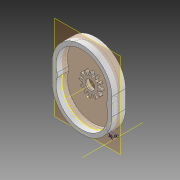
# Autodesk Inventor part: housing
Saved by Autodesk Inventor 2020 (Build 240168000, 168)
## iProperties
Created: 2020-11-24
Part Number: housing
Material: Generic
Document SubType Name: Modeling
Designer: DDeGo
Density: 1 g/cm^3
Appearance: Default
Author: DDeGo
Autodesk Inventor part; units mm, degrees
(part 1 of 10)
ref_plane "YZ Plane" through (0, 0, 0) normal (1, 0, 0) x (0, 1, 0)
ref_plane "XZ Plane" through (0, 0, 0) normal (0, 1, 0) x (-1, 0, 0)
ref_plane "XY Plane" through (0, 0, 0) normal (0, 0, 1) x (1, 0, 0)
sketch "Block1" plane through (0, 0, 0) normal (0, 0, 1) x (1, 0, 0)
  arc A0 (4.126, -4.0048) -> (4.8225, -3.1314) centre (0, 0) ccw
  line L0 (4.8225, -3.1314) -> (5.5168, -3.5822)
  spline S0 degree 5 poles (5.5174, -3.5826) (5.5175, -3.5826) (5.5176, -3.5827) (5.5178, -3.5828) (5.5181, -3.583) (5.5186, -3.5833) (5.5191, -3.5837) (5.5197, -3.584) (5.5204, -3.5844) (5.5211, -3.5849) (5.522, -3.5854) (5.5228, -3.5859) (5.5238, -3.5864) (5.5248, -3.587) (5.5259, -3.5877) (5.5271, -3.5883) (5.5283, -3.589) (5.5296, -3.5897) (5.531, -3.5905) (5.5324, -3.5913) (5.5339, -3.5921) (5.5355, -3.593) (5.5371, -3.5938) (5.5388, -3.5947) (5.5405, -3.5957) (5.5424, -3.5966) (5.5442, -3.5976) (5.5462, -3.5986) (5.5482, -3.5996) (5.5503, -3.6007) (5.5524, -3.6018) (5.5546, -3.6029) (5.5569, -3.604) (5.5592, -3.6051) (5.5616, -3.6063) (5.5645, -3.6077) (5.5676, -3.6092) (5.5707, -3.6106) (5.5749, -3.6126) (5.5805, -3.6152) (5.5857, -3.6176) (5.5912, -3.62) (5.5968, -3.6224) (5.6032, -3.6252) (5.6085, -3.6275) (5.614, -3.6298) (5.6196, -3.6321) (5.6269, -3.635) (5.632, -3.6371) (5.6373, -3.6392) (5.6435, -3.6416) (5.6499, -3.6441) (5.6547, -3.6459) (5.6596, -3.6477) (5.6671, -3.6505) (5.6739, -3.653) (5.6808, -3.6555) (5.6879, -3.658) (5.697, -3.6611) (5.7035, -3.6633) (5.71, -3.6656) (5.7167, -3.6678) (5.7254, -3.6706) (5.7322, -3.6728) (5.7392, -3.675) (5.7463, -3.6772) (5.7556, -3.6801) (5.7628, -3.6823) (5.7702, -3.6845) (5.7788, -3.687) (5.7875, -3.6895) (5.7941, -3.6914) (5.8019, -3.6935) (5.8098, -3.6957) (5.8166, -3.6976) (5.8246, -3.6997) (5.8328, -3.7019) (5.8398, -3.7037) (5.8481, -3.7058) (5.8565, -3.7079) (5.8638, -3.7097) (5.8723, -3.7118) (5.881, -3.7138) (5.8885, -3.7156) (5.8973, -3.7176) (5.9062, -3.7196) (5.9139, -3.7214) (5.9229, -3.7233) (5.9321, -3.7253) (5.94, -3.727) (5.9493, -3.7289) (5.9586, -3.7308) (5.9667, -3.7324) (5.9763, -3.7343) (5.9859, -3.7361) (5.9942, -3.7377) (6.004, -3.7395) (6.0138, -3.7413) (6.0223, -3.7428) (6.0323, -3.7445) (6.0424, -3.7462) (6.0511, -3.7477) (6.0613, -3.7493) (6.0716, -3.751) (6.0805, -3.7523) (6.091, -3.7539) (6.1015, -3.7555) (6.1106, -3.7568) (6.1212, -3.7582) (6.132, -3.7597) (6.1412, -3.7609) (6.1521, -3.7623) (6.1631, -3.7637) (6.1725, -3.7649) (6.1836, -3.7662) (6.1947, -3.7675) (6.2044, -3.7685) (6.2157, -3.7697) (6.227, -3.7709) (6.2368, -3.7719) (6.2483, -3.773) (6.2599, -3.7741) (6.2699, -3.775) (6.2816, -3.776) (6.2933, -3.777) (6.3035, -3.7778) (6.3153, -3.7787) (6.3273, -3.7796) (6.3376, -3.7803) (6.3497, -3.7811) (6.3618, -3.7818) (6.3723, -3.7824) (6.3846, -3.7831) (6.3969, -3.7838) (6.4075, -3.7843) (6.42, -3.7848) (6.4325, -3.7854) (6.4433, -3.7858) (6.4559, -3.7862) (6.4686, -3.7866) (6.4796, -3.7869) (6.4924, -3.7872) (6.5053, -3.7875) (6.5164, -3.7877) (6.5294, -3.7879) (6.5424, -3.788) (6.5536, -3.7881) (6.5649, -3.7882) (6.5781, -3.7882) (6.5895, -3.7882) (6.6009, -3.7881) (6.6143, -3.788) (6.6277, -3.7879) (6.6393, -3.7877) (6.6547, -3.7874) (6.6703, -3.7871) (6.6839, -3.7868) (6.6996, -3.7863) (6.7154, -3.7858) (6.7272, -3.7853) (6.7392, -3.7849) (6.7511, -3.7843) (6.7611, -3.7839) (6.7711, -3.7834) (6.7811, -3.7829) (6.7912, -3.7824) (6.8013, -3.7818) (6.8114, -3.7812) (6.8215, -3.7806) (6.8317, -3.78) (6.8419, -3.7793) (6.8521, -3.7787) (6.8624, -3.7779) (6.8726, -3.7772) (6.8829, -3.7764) (6.8933, -3.7756) (6.9036, -3.7748) (6.914, -3.774) (6.9244, -3.7731) (6.9348, -3.7722) (6.9452, -3.7713) (6.9557, -3.7703) (6.9662, -3.7693) (6.9767, -3.7683) (6.9873, -3.7673) (6.9979, -3.7662) (7.0148, -3.7644) (7.0297, -3.7628) (7.0425, -3.7614) (7.0532, -3.7602) (7.0618, -3.7592) knots 0 0 0 0 0 0 0.004167 0.008333 0.0125 0.016667 0.020833 0.025 0.029167 0.033333 0.0375 0.041667 0.045833 0.05 0.054167 0.058333 0.0625 0.066667 0.070833 0.075 0.079167 0.083333 0.0875 0.091667 0.095833 0.1 0.104167 0.108333 0.1125 0.116667 0.120833 0.125 0.129167 0.133333 0.1375 0.141667 0.15 0.154167 0.158333 0.170833 0.183333 0.1875 0.191667 0.195833 0.2125 0.216667 0.220833 0.225 0.2375 0.241667 0.245833 0.254167 0.258333 0.2625 0.266667 0.283333 0.2875 0.291667 0.295833 0.308333 0.3125 0.316667 0.320833 0.333333 0.3375 0.341667 0.345833 0.358333 0.3625 0.366667 0.375 0.379167 0.383333 0.391667 0.395833 0.4 0.408333 0.4125 0.416667 0.425 0.429167 0.433333 0.441667 0.445833 0.45 0.458333 0.4625 0.466667 0.475 0.479167 0.483333 0.491667 0.495833 0.5 0.508333 0.5125 0.516667 0.525 0.529167 0.533333 0.541667 0.545833 0.55 0.558333 0.5625 0.566667 0.575 0.579167 0.583333 0.591667 0.595833 0.6 0.608333 0.6125 0.616667 0.625 0.629167 0.633333 0.641667 0.645833 0.65 0.658333 0.6625 0.666667 0.675 0.679167 0.683333 0.691667 0.695833 0.7 0.708333 0.7125 0.716667 0.725 0.729167 0.733333 0.741667 0.745833 0.75 0.758333 0.7625 0.766667 0.775 0.779167 0.783333 0.791667 0.795833 0.8 0.804167 0.8125 0.816667 0.820833 0.829167 0.833333 0.8375 0.85 0.854167 0.858333 0.866667 0.870833 0.875 0.879167 0.883333 0.8875 0.891667 0.895833 0.9 0.904167 0.908333 0.9125 0.916667 0.920833 0.925 0.929167 0.933333 0.9375 0.941667 0.945833 0.95 0.954167 0.958333 0.9625 0.966667 0.970833 0.975 0.979167 0.983333 1 1 1 1 1 1
  arc A1 (7.0618, -3.7592) -> (7.342, -3.1773) centre (0, 0) ccw
  line L1 (6.241, -2.08) -> (6.2404, -2.0798)
  line L2 (6.2404, -2.0798) -> (5.455, -1.818)
  arc A2 (5.455, -1.818) -> (5.7036, -0.7289) centre (0, 0) ccw
  spline S1 degree 5 poles (7.342, -3.1773) (7.3386, -3.1718) (7.334, -3.1645) (7.3283, -3.1554) (7.3214, -3.1445) (7.3134, -3.1319) (7.3076, -3.123) (7.3019, -3.114) (7.2961, -3.1051) (7.2903, -3.0963) (7.2846, -3.0875) (7.2788, -3.0787) (7.273, -3.0699) (7.2672, -3.0612) (7.2614, -3.0525) (7.2556, -3.0439) (7.2498, -3.0353) (7.244, -3.0267) (7.2381, -3.0182) (7.2323, -3.0097) (7.2265, -3.0012) (7.2207, -2.9928) (7.2148, -2.9844) (7.209, -2.9761) (7.2031, -2.9678) (7.1973, -2.9595) (7.1914, -2.9513) (7.1856, -2.9431) (7.1797, -2.9349) (7.1738, -2.9268) (7.1668, -2.9171) (7.1597, -2.9075) (7.1527, -2.8979) (7.1456, -2.8883) (7.1362, -2.8757) (7.128, -2.8647) (7.1197, -2.8538) (7.1115, -2.843) (7.1021, -2.8307) (7.095, -2.8216) (7.0855, -2.8094) (7.0761, -2.7974) (7.0667, -2.7855) (7.0572, -2.7737) (7.0478, -2.762) (7.0407, -2.7533) (7.0325, -2.7431) (7.0242, -2.7331) (7.0172, -2.7246) (7.0101, -2.7161) (6.9995, -2.7034) (6.9901, -2.6923) (6.9807, -2.6813) (6.9713, -2.6704) (6.9596, -2.6569) (6.9514, -2.6475) (6.9432, -2.6382) (6.935, -2.629) (6.9233, -2.6159) (6.914, -2.6056) (6.9046, -2.5954) (6.8953, -2.5853) (6.8849, -2.5741) (6.878, -2.5666) (6.871, -2.5593) (6.8629, -2.5507) (6.8548, -2.5423) (6.8479, -2.5351) (6.8399, -2.5268) (6.8319, -2.5185) (6.825, -2.5115) (6.817, -2.5034) (6.809, -2.4954) (6.8022, -2.4886) (6.7942, -2.4807) (6.7863, -2.4729) (6.7795, -2.4663) (6.7717, -2.4587) (6.7638, -2.4511) (6.7571, -2.4447) (6.7493, -2.4372) (6.7415, -2.4299) (6.7348, -2.4237) (6.727, -2.4164) (6.7193, -2.4093) (6.7127, -2.4033) (6.705, -2.3963) (6.6974, -2.3894) (6.6908, -2.3835) (6.6832, -2.3768) (6.6757, -2.3701) (6.6692, -2.3644) (6.6617, -2.3579) (6.6542, -2.3514) (6.6479, -2.346) (6.6404, -2.3396) (6.6331, -2.3334) (6.6268, -2.3281) (6.6194, -2.322) (6.6122, -2.316) (6.606, -2.3109) (6.5988, -2.3051) (6.5916, -2.2993) (6.5855, -2.2944) (6.5784, -2.2888) (6.5713, -2.2832) (6.5653, -2.2785) (6.5583, -2.2731) (6.5514, -2.2677) (6.5455, -2.2632) (6.5387, -2.258) (6.5319, -2.2529) (6.5261, -2.2486) (6.5194, -2.2436) (6.5127, -2.2387) (6.507, -2.2346) (6.5005, -2.2298) (6.4939, -2.2251) (6.4884, -2.2212) (6.482, -2.2167) (6.4756, -2.2122) (6.4702, -2.2085) (6.464, -2.2042) (6.4578, -2.1999) (6.4525, -2.1964) (6.4464, -2.1923) (6.4404, -2.1883) (6.4352, -2.1849) (6.4293, -2.181) (6.4235, -2.1772) (6.4185, -2.174) (6.4128, -2.1704) (6.4071, -2.1668) (6.4023, -2.1638) (6.3968, -2.1604) (6.3913, -2.157) (6.3867, -2.1542) (6.3814, -2.151) (6.3761, -2.1478) (6.3717, -2.1452) (6.3665, -2.1422) (6.3615, -2.1393) (6.3573, -2.1368) (6.3524, -2.134) (6.3476, -2.1313) (6.3435, -2.129) (6.3388, -2.1265) (6.3343, -2.1239) (6.3304, -2.1219) (6.326, -2.1195) (6.3217, -2.1172) (6.3181, -2.1153) (6.3145, -2.1134) (6.3099, -2.111) (6.3059, -2.109) (6.302, -2.107) (6.2983, -2.1052) (6.2946, -2.1034) (6.2921, -2.1021) (6.2896, -2.1009) (6.2871, -2.0997) (6.2847, -2.0986) (6.2824, -2.0975) (6.2801, -2.0964) (6.2778, -2.0954) (6.2757, -2.0944) (6.2736, -2.0934) (6.2715, -2.0925) (6.2695, -2.0916) (6.2675, -2.0907) (6.2657, -2.0899) (6.2638, -2.0891) (6.2621, -2.0884) (6.2604, -2.0876) (6.2587, -2.0869) (6.2572, -2.0863) (6.2557, -2.0856) (6.2542, -2.0851) (6.2529, -2.0845) (6.2515, -2.084) (6.2503, -2.0835) (6.2491, -2.083) (6.248, -2.0826) (6.247, -2.0822) (6.246, -2.0818) (6.2451, -2.0815) (6.2443, -2.0812) (6.2436, -2.0809) (6.2429, -2.0806) (6.2422, -2.0804) (6.2417, -2.0802) (6.2414, -2.0801) (6.2412, -2.08) (6.241, -2.08) knots -1 -1 -1 -1 -1 -1 -0.9875 -0.983333 -0.979167 -0.975 -0.970833 -0.966667 -0.9625 -0.958333 -0.954167 -0.95 -0.945833 -0.941667 -0.9375 -0.933333 -0.929167 -0.925 -0.920833 -0.916667 -0.9125 -0.908333 -0.904167 -0.9 -0.895833 -0.891667 -0.8875 -0.883333 -0.879167 -0.875 -0.870833 -0.8625 -0.858333 -0.854167 -0.85 -0.8375 -0.833333 -0.829167 -0.825 -0.816667 -0.8125 -0.8 -0.795833 -0.791667 -0.783333 -0.779167 -0.775 -0.766667 -0.7625 -0.758333 -0.754167 -0.7375 -0.733333 -0.729167 -0.725 -0.7125 -0.708333 -0.704167 -0.7 -0.683333 -0.679167 -0.675 -0.670833 -0.6625 -0.658333 -0.654167 -0.645833 -0.641667 -0.6375 -0.629167 -0.625 -0.620833 -0.6125 -0.608333 -0.604167 -0.595833 -0.591667 -0.5875 -0.579167 -0.575 -0.570833 -0.5625 -0.558333 -0.554167 -0.545833 -0.541667 -0.5375 -0.529167 -0.525 -0.520833 -0.5125 -0.508333 -0.504167 -0.495833 -0.491667 -0.4875 -0.479167 -0.475 -0.470833 -0.4625 -0.458333 -0.454167 -0.445833 -0.441667 -0.4375 -0.429167 -0.425 -0.420833 -0.4125 -0.408333 -0.404167 -0.395833 -0.391667 -0.3875 -0.379167 -0.375 -0.370833 -0.3625 -0.358333 -0.354167 -0.345833 -0.341667 -0.3375 -0.329167 -0.325 -0.320833 -0.3125 -0.308333 -0.304167 -0.295833 -0.291667 -0.2875 -0.279167 -0.275 -0.270833 -0.2625 -0.258333 -0.254167 -0.245833 -0.241667 -0.2375 -0.229167 -0.225 -0.220833 -0.2125 -0.208333 -0.204167 -0.195833 -0.191667 -0.1875 -0.179167 -0.175 -0.170833 -0.166667 -0.154167 -0.15 -0.145833 -0.141667 -0.1375 -0.133333 -0.129167 -0.125 -0.120833 -0.116667 -0.1125 -0.108333 -0.104167 -0.1 -0.095833 -0.091667 -0.0875 -0.083333 -0.079167 -0.075 -0.070833 -0.066667 -0.0625 -0.058333 -0.054167 -0.05 -0.045833 -0.041667 -0.0375 -0.033333 -0.029167 -0.025 -0.020833 -0.016667 -0.0125 -0.008333 0 0 0 0 0 0
  line L3 (5.5168, -3.5822) -> (5.5174, -3.5826)
  line L4 (4.72, 4.5814) -> (4.7205, 4.5819)
  line L5 (4.126, 4.0048) -> (4.72, 4.5814)
  spline S2 degree 5 poles (4.7205, 4.5819) (4.7206, 4.5819) (4.7207, 4.582) (4.7208, 4.5822) (4.7211, 4.5824) (4.7215, 4.5828) (4.7219, 4.5833) (4.7224, 4.5838) (4.723, 4.5844) (4.7236, 4.585) (4.7242, 4.5857) (4.7249, 4.5864) (4.7257, 4.5872) (4.7265, 4.5881) (4.7273, 4.589) (4.7282, 4.59) (4.7292, 4.5911) (4.7302, 4.5922) (4.7312, 4.5933) (4.7323, 4.5946) (4.7335, 4.5958) (4.7346, 4.5972) (4.7358, 4.5986) (4.7371, 4.6) (4.7384, 4.6015) (4.7397, 4.6031) (4.7411, 4.6047) (4.7425, 4.6064) (4.744, 4.6081) (4.7455, 4.6099) (4.747, 4.6117) (4.7485, 4.6136) (4.7501, 4.6156) (4.7518, 4.6176) (4.7534, 4.6197) (4.7555, 4.6222) (4.7576, 4.6248) (4.7597, 4.6276) (4.7626, 4.6313) (4.7663, 4.6361) (4.7698, 4.6407) (4.7734, 4.6455) (4.777, 4.6504) (4.7812, 4.6561) (4.7846, 4.6607) (4.788, 4.6655) (4.7915, 4.6705) (4.796, 4.6769) (4.7992, 4.6815) (4.8024, 4.6862) (4.8057, 4.691) (4.8104, 4.698) (4.8142, 4.7038) (4.8181, 4.7097) (4.822, 4.7157) (4.827, 4.7234) (4.8305, 4.729) (4.834, 4.7346) (4.8376, 4.7403) (4.8422, 4.7478) (4.8458, 4.7537) (4.8494, 4.7598) (4.8531, 4.7659) (4.8584, 4.7748) (4.8627, 4.7821) (4.8669, 4.7895) (4.8712, 4.7971) (4.8767, 4.8067) (4.8805, 4.8135) (4.8843, 4.8204) (4.8881, 4.8274) (4.8931, 4.8366) (4.897, 4.8438) (4.9008, 4.8511) (4.9047, 4.8585) (4.9097, 4.8682) (4.9136, 4.8758) (4.9176, 4.8835) (4.9221, 4.8924) (4.9265, 4.9014) (4.9299, 4.9083) (4.9333, 4.9152) (4.9378, 4.9245) (4.9418, 4.9327) (4.9457, 4.9411) (4.9502, 4.9507) (4.9547, 4.9605) (4.9581, 4.9679) (4.9621, 4.9766) (4.966, 4.9853) (4.9694, 4.9929) (4.9733, 5.0019) (4.9773, 5.0109) (4.9806, 5.0187) (4.9846, 5.0279) (4.9885, 5.0372) (4.9918, 5.0452) (4.9957, 5.0546) (4.9996, 5.0641) (5.003, 5.0723) (5.0069, 5.082) (5.0107, 5.0917) (5.014, 5.1001) (5.0179, 5.11) (5.0217, 5.12) (5.025, 5.1286) (5.0288, 5.1387) (5.0327, 5.1489) (5.0359, 5.1577) (5.0397, 5.1681) (5.0434, 5.1785) (5.0467, 5.1875) (5.0504, 5.1981) (5.0541, 5.2087) (5.0573, 5.2179) (5.061, 5.2287) (5.0646, 5.2396) (5.0678, 5.2489) (5.0714, 5.26) (5.075, 5.2711) (5.0781, 5.2806) (5.0817, 5.2918) (5.0852, 5.3032) (5.0883, 5.3129) (5.0918, 5.3244) (5.0953, 5.3359) (5.0982, 5.3458) (5.1017, 5.3575) (5.1051, 5.3692) (5.108, 5.3793) (5.1114, 5.3912) (5.1147, 5.4031) (5.1176, 5.4134) (5.1209, 5.4255) (5.1242, 5.4376) (5.1269, 5.4481) (5.1311, 5.4638) (5.1352, 5.4798) (5.1388, 5.494) (5.1423, 5.5083) (5.1467, 5.5264) (5.1498, 5.5391) (5.1528, 5.5519) (5.1557, 5.5647) (5.1591, 5.5795) (5.1616, 5.5906) (5.1645, 5.6037) (5.1673, 5.6168) (5.1701, 5.63) (5.1729, 5.6432) (5.1757, 5.6565) (5.178, 5.668) (5.1803, 5.6795) (5.1833, 5.6949) (5.1859, 5.7085) (5.1885, 5.7221) (5.191, 5.7358) (5.1935, 5.7496) (5.1953, 5.7594) (5.197, 5.7693) (5.1987, 5.7793) (5.2004, 5.7892) (5.2021, 5.7992) (5.2038, 5.8092) (5.2054, 5.8193) (5.207, 5.8294) (5.2087, 5.8395) (5.2102, 5.8496) (5.2118, 5.8598) (5.2133, 5.87) (5.2149, 5.8803) (5.2164, 5.8905) (5.2178, 5.9008) (5.2193, 5.9112) (5.2207, 5.9215) (5.2222, 5.9319) (5.2236, 5.9424) (5.2249, 5.9528) (5.2263, 5.9633) (5.2276, 5.9738) (5.2289, 5.9844) (5.231, 6.0013) (5.2327, 6.0161) (5.2342, 6.0289) (5.2354, 6.0396) (5.2363, 6.0482) knots 0 0 0 0 0 0 0.004167 0.008333 0.0125 0.016667 0.020833 0.025 0.029167 0.033333 0.0375 0.041667 0.045833 0.05 0.054167 0.058333 0.0625 0.066667 0.070833 0.075 0.079167 0.083333 0.0875 0.091667 0.095833 0.1 0.104167 0.108333 0.1125 0.116667 0.120833 0.125 0.129167 0.133333 0.1375 0.141667 0.15 0.154167 0.158333 0.170833 0.183333 0.1875 0.191667 0.195833 0.2125 0.216667 0.220833 0.225 0.2375 0.241667 0.245833 0.25 0.266667 0.270833 0.275 0.279167 0.291667 0.295833 0.3 0.304167 0.316667 0.320833 0.325 0.329167 0.345833 0.35 0.354167 0.358333 0.370833 0.375 0.379167 0.383333 0.395833 0.4 0.404167 0.408333 0.420833 0.425 0.429167 0.4375 0.441667 0.445833 0.45 0.4625 0.466667 0.470833 0.479167 0.483333 0.4875 0.495833 0.5 0.504167 0.5125 0.516667 0.520833 0.529167 0.533333 0.5375 0.545833 0.55 0.554167 0.5625 0.566667 0.570833 0.579167 0.583333 0.5875 0.595833 0.6 0.604167 0.6125 0.616667 0.620833 0.629167 0.633333 0.6375 0.645833 0.65 0.654167 0.6625 0.666667 0.670833 0.679167 0.683333 0.6875 0.695833 0.7 0.704167 0.7125 0.716667 0.720833 0.729167 0.733333 0.7375 0.745833 0.75 0.754167 0.770833 0.775 0.779167 0.783333 0.795833 0.8 0.804167 0.808333 0.816667 0.820833 0.829167 0.833333 0.8375 0.845833 0.85 0.854167 0.858333 0.870833 0.875 0.879167 0.883333 0.8875 0.891667 0.895833 0.9 0.904167 0.908333 0.9125 0.916667 0.920833 0.925 0.929167 0.933333 0.9375 0.941667 0.945833 0.95 0.954167 0.958333 0.9625 0.966667 0.970833 0.975 0.979167 0.983333 1 1 1 1 1 1
  arc A3 (5.2363, 6.0482) -> (4.7314, 6.4509) centre (0, 0) ccw
  line L6 (3.4166, 5.6217) -> (3.4162, 5.6212)
  spline S3 degree 5 poles (4.7314, 6.4509) (4.7253, 6.4488) (4.7171, 6.4459) (4.707, 6.4424) (4.6949, 6.4381) (4.6808, 6.4331) (4.6708, 6.4295) (4.6608, 6.4258) (4.6508, 6.4222) (4.6409, 6.4186) (4.631, 6.4149) (4.6212, 6.4112) (4.6114, 6.4075) (4.6016, 6.4038) (4.5918, 6.4001) (4.5821, 6.3963) (4.5724, 6.3926) (4.5628, 6.3888) (4.5532, 6.3851) (4.5436, 6.3813) (4.534, 6.3775) (4.5245, 6.3737) (4.5151, 6.3698) (4.5056, 6.366) (4.4962, 6.3621) (4.4869, 6.3583) (4.4775, 6.3544) (4.4682, 6.3505) (4.459, 6.3466) (4.4498, 6.3427) (4.4406, 6.3388) (4.4277, 6.3333) (4.415, 6.3277) (4.4023, 6.3222) (4.3898, 6.3166) (4.3737, 6.3094) (4.3559, 6.3014) (4.3383, 6.2933) (4.3209, 6.2852) (4.3036, 6.277) (4.2865, 6.2688) (4.2745, 6.2631) (4.2627, 6.2573) (4.2509, 6.2516) (4.2359, 6.2441) (4.2243, 6.2383) (4.2128, 6.2325) (4.1997, 6.2258) (4.1867, 6.2191) (4.177, 6.2141) (4.1658, 6.2082) (4.1547, 6.2023) (4.1452, 6.1972) (4.1342, 6.1913) (4.1233, 6.1854) (4.114, 6.1803) (4.1032, 6.1744) (4.0925, 6.1685) (4.0834, 6.1634) (4.0728, 6.1574) (4.0623, 6.1514) (4.0534, 6.1463) (4.043, 6.1404) (4.0328, 6.1344) (4.024, 6.1292) (4.0139, 6.1233) (4.0039, 6.1173) (3.9953, 6.1121) (3.9854, 6.1061) (3.9756, 6.1002) (3.9673, 6.095) (3.9576, 6.089) (3.948, 6.083) (3.9398, 6.0779) (3.9317, 6.0727) (3.9197, 6.065) (3.9091, 6.0582) (3.8986, 6.0514) (3.8882, 6.0445) (3.8754, 6.036) (3.8665, 6.03) (3.8577, 6.0241) (3.849, 6.0181) (3.838, 6.0105) (3.8294, 6.0045) (3.821, 5.9986) (3.8126, 5.9927) (3.8008, 5.9843) (3.7915, 5.9776) (3.7823, 5.9708) (3.7732, 5.9642) (3.762, 5.9558) (3.7542, 5.95) (3.7465, 5.9442) (3.7389, 5.9384) (3.7293, 5.931) (3.7219, 5.9253) (3.7146, 5.9196) (3.7074, 5.9139) (3.6982, 5.9066) (3.6912, 5.9009) (3.6842, 5.8953) (3.6764, 5.8889) (3.6687, 5.8825) (3.663, 5.8778) (3.6564, 5.8723) (3.6499, 5.8668) (3.6444, 5.8621) (3.638, 5.8567) (3.6318, 5.8513) (3.6265, 5.8466) (3.6204, 5.8413) (3.6144, 5.836) (3.6093, 5.8315) (3.6035, 5.8262) (3.5977, 5.821) (3.5929, 5.8166) (3.5873, 5.8114) (3.5818, 5.8063) (3.5771, 5.802) (3.5718, 5.7969) (3.5665, 5.792) (3.5621, 5.7877) (3.557, 5.7828) (3.552, 5.778) (3.5478, 5.7738) (3.5429, 5.7691) (3.5382, 5.7643) (3.5342, 5.7603) (3.5296, 5.7557) (3.5251, 5.7511) (3.5214, 5.7472) (3.517, 5.7427) (3.5128, 5.7383) (3.5092, 5.7346) (3.5052, 5.7302) (3.5012, 5.726) (3.4979, 5.7224) (3.494, 5.7182) (3.4903, 5.7141) (3.4872, 5.7107) (3.4837, 5.7067) (3.4802, 5.7028) (3.4773, 5.6995) (3.474, 5.6958) (3.4708, 5.6921) (3.4681, 5.689) (3.4655, 5.6859) (3.4622, 5.6819) (3.4593, 5.6785) (3.4565, 5.6752) (3.4539, 5.6719) (3.4513, 5.6687) (3.4495, 5.6665) (3.4478, 5.6644) (3.4461, 5.6622) (3.4445, 5.6602) (3.4429, 5.6581) (3.4413, 5.6561) (3.4398, 5.6542) (3.4383, 5.6523) (3.4369, 5.6504) (3.4356, 5.6486) (3.4342, 5.6469) (3.433, 5.6452) (3.4317, 5.6435) (3.4306, 5.6419) (3.4294, 5.6404) (3.4283, 5.6389) (3.4273, 5.6374) (3.4263, 5.6361) (3.4254, 5.6347) (3.4245, 5.6335) (3.4236, 5.6322) (3.4228, 5.6311) (3.4221, 5.63) (3.4213, 5.6289) (3.4207, 5.628) (3.4201, 5.627) (3.4195, 5.6262) (3.419, 5.6254) (3.4185, 5.6247) (3.418, 5.624) (3.4176, 5.6234) (3.4172, 5.6228) (3.417, 5.6223) (3.4168, 5.622) (3.4166, 5.6218) (3.4166, 5.6217) knots -1 -1 -1 -1 -1 -1 -0.9875 -0.983333 -0.979167 -0.975 -0.970833 -0.966667 -0.9625 -0.958333 -0.954167 -0.95 -0.945833 -0.941667 -0.9375 -0.933333 -0.929167 -0.925 -0.920833 -0.916667 -0.9125 -0.908333 -0.904167 -0.9 -0.895833 -0.891667 -0.8875 -0.883333 -0.879167 -0.875 -0.870833 -0.866667 -0.854167 -0.85 -0.845833 -0.841667 -0.829167 -0.8125 -0.808333 -0.804167 -0.8 -0.7875 -0.783333 -0.779167 -0.775 -0.7625 -0.758333 -0.754167 -0.745833 -0.741667 -0.7375 -0.729167 -0.725 -0.720833 -0.7125 -0.708333 -0.704167 -0.695833 -0.691667 -0.6875 -0.679167 -0.675 -0.670833 -0.6625 -0.658333 -0.654167 -0.645833 -0.641667 -0.6375 -0.629167 -0.625 -0.620833 -0.6125 -0.608333 -0.604167 -0.6 -0.583333 -0.579167 -0.575 -0.570833 -0.558333 -0.554167 -0.55 -0.545833 -0.533333 -0.529167 -0.525 -0.520833 -0.504167 -0.5 -0.495833 -0.491667 -0.479167 -0.475 -0.470833 -0.466667 -0.454167 -0.45 -0.445833 -0.441667 -0.429167 -0.425 -0.420833 -0.4125 -0.408333 -0.404167 -0.395833 -0.391667 -0.3875 -0.379167 -0.375 -0.370833 -0.3625 -0.358333 -0.354167 -0.345833 -0.341667 -0.3375 -0.329167 -0.325 -0.320833 -0.3125 -0.308333 -0.304167 -0.295833 -0.291667 -0.2875 -0.279167 -0.275 -0.270833 -0.2625 -0.258333 -0.254167 -0.245833 -0.241667 -0.2375 -0.229167 -0.225 -0.220833 -0.2125 -0.208333 -0.204167 -0.195833 -0.191667 -0.1875 -0.179167 -0.175 -0.170833 -0.166667 -0.154167 -0.15 -0.145833 -0.141667 -0.1375 -0.133333 -0.129167 -0.125 -0.120833 -0.116667 -0.1125 -0.108333 -0.104167 -0.1 -0.095833 -0.091667 -0.0875 -0.083333 -0.079167 -0.075 -0.070833 -0.066667 -0.0625 -0.058333 -0.054167 -0.05 -0.045833 -0.041667 -0.0375 -0.033333 -0.029167 -0.025 -0.020833 -0.016667 -0.0125 -0.008333 0 0 0 0 0 0
  arc A4 (2.9863, 4.9137) -> (1.9798, 5.3984) centre (0, 0) ccw
  line L7 (2.2648, 6.1757) -> (2.265, 6.1763)
  line L8 (1.9798, 5.3984) -> (2.2648, 6.1757)
  line L9 (0.6391, 6.5474) -> (0.639, 6.5467)
  spline S4 degree 5 poles (2.265, 6.1763) (2.2651, 6.1763) (2.2651, 6.1765) (2.2652, 6.1767) (2.2653, 6.177) (2.2655, 6.1776) (2.2657, 6.1782) (2.2659, 6.1788) (2.2662, 6.1796) (2.2664, 6.1804) (2.2667, 6.1813) (2.267, 6.1823) (2.2674, 6.1834) (2.2677, 6.1845) (2.2681, 6.1857) (2.2685, 6.187) (2.2689, 6.1883) (2.2693, 6.1898) (2.2697, 6.1913) (2.2702, 6.1928) (2.2706, 6.1945) (2.2711, 6.1962) (2.2716, 6.198) (2.2721, 6.1998) (2.2726, 6.2017) (2.2732, 6.2037) (2.2737, 6.2058) (2.2742, 6.2079) (2.2748, 6.2101) (2.2754, 6.2123) (2.2759, 6.2147) (2.2765, 6.2171) (2.2771, 6.2195) (2.2777, 6.222) (2.2783, 6.2246) (2.279, 6.2278) (2.2798, 6.2311) (2.2805, 6.2344) (2.2815, 6.2391) (2.2828, 6.2451) (2.2839, 6.2507) (2.2851, 6.2565) (2.2862, 6.2625) (2.2875, 6.2694) (2.2885, 6.2751) (2.2895, 6.281) (2.2906, 6.287) (2.2918, 6.2947) (2.2927, 6.3002) (2.2935, 6.3058) (2.2944, 6.3115) (2.2956, 6.3199) (2.2966, 6.3268) (2.2975, 6.3338) (2.2984, 6.3409) (2.2995, 6.35) (2.3003, 6.3565) (2.301, 6.3631) (2.3017, 6.3698) (2.3027, 6.3786) (2.3033, 6.3855) (2.304, 6.3925) (2.3047, 6.4007) (2.3055, 6.4089) (2.306, 6.4152) (2.3065, 6.4216) (2.3072, 6.4312) (2.3078, 6.4399) (2.3083, 6.4488) (2.3089, 6.4577) (2.3095, 6.4691) (2.3099, 6.4771) (2.3102, 6.4853) (2.3106, 6.4935) (2.3109, 6.5042) (2.3112, 6.5127) (2.3114, 6.5212) (2.3117, 6.531) (2.3118, 6.541) (2.312, 6.5485) (2.312, 6.5561) (2.3121, 6.5663) (2.3121, 6.5754) (2.3121, 6.5845) (2.3121, 6.595) (2.312, 6.6056) (2.3119, 6.6136) (2.3117, 6.6231) (2.3115, 6.6326) (2.3113, 6.6408) (2.311, 6.6504) (2.3107, 6.6602) (2.3104, 6.6686) (2.31, 6.6785) (2.3096, 6.6884) (2.3092, 6.697) (2.3087, 6.7071) (2.3082, 6.7172) (2.3077, 6.726) (2.307, 6.7363) (2.3064, 6.7466) (2.3057, 6.7556) (2.305, 6.766) (2.3042, 6.7766) (2.3035, 6.7857) (2.3026, 6.7964) (2.3016, 6.8071) (2.3008, 6.8164) (2.2998, 6.8272) (2.2987, 6.8382) (2.2978, 6.8476) (2.2966, 6.8587) (2.2954, 6.8698) (2.2944, 6.8794) (2.2931, 6.8906) (2.2917, 6.9019) (2.2905, 6.9116) (2.2891, 6.9231) (2.2876, 6.9345) (2.2863, 6.9444) (2.2847, 6.956) (2.2831, 6.9676) (2.2817, 6.9777) (2.2799, 6.9894) (2.2782, 7.0012) (2.2766, 7.0114) (2.2747, 7.0233) (2.2728, 7.0353) (2.2711, 7.0456) (2.2691, 7.0577) (2.267, 7.0698) (2.2651, 7.0802) (2.263, 7.0925) (2.2607, 7.1048) (2.2588, 7.1153) (2.2564, 7.1277) (2.254, 7.1402) (2.2519, 7.1509) (2.2494, 7.1634) (2.2469, 7.176) (2.2446, 7.1868) (2.2412, 7.2031) (2.2377, 7.2195) (2.2344, 7.2341) (2.2311, 7.2488) (2.2265, 7.2691) (2.223, 7.2839) (2.2195, 7.2988) (2.2158, 7.3138) (2.2117, 7.3307) (2.2088, 7.342) (2.2059, 7.3533) (2.2025, 7.3666) (2.1991, 7.3799) (2.196, 7.3913) (2.193, 7.4028) (2.1898, 7.4143) (2.1872, 7.4239) (2.1845, 7.4336) (2.1818, 7.4432) (2.1791, 7.4529) (2.1764, 7.4626) (2.1736, 7.4723) (2.1708, 7.482) (2.1679, 7.4918) (2.165, 7.5015) (2.1621, 7.5113) (2.1592, 7.5211) (2.1562, 7.531) (2.1532, 7.5408) (2.1501, 7.5507) (2.1471, 7.5606) (2.144, 7.5705) (2.1408, 7.5804) (2.1377, 7.5904) (2.1345, 7.6003) (2.1312, 7.6103) (2.128, 7.6203) (2.1247, 7.6303) (2.1213, 7.6403) (2.118, 7.6504) (2.1146, 7.6605) (2.1091, 7.6766) (2.1042, 7.6907) (2.1, 7.7029) (2.0964, 7.7131) (2.0935, 7.7212) knots 0 0 0 0 0 0 0.004167 0.008333 0.0125 0.016667 0.020833 0.025 0.029167 0.033333 0.0375 0.041667 0.045833 0.05 0.054167 0.058333 0.0625 0.066667 0.070833 0.075 0.079167 0.083333 0.0875 0.091667 0.095833 0.1 0.104167 0.108333 0.1125 0.116667 0.120833 0.125 0.129167 0.133333 0.1375 0.141667 0.15 0.154167 0.158333 0.170833 0.183333 0.1875 0.191667 0.195833 0.2125 0.216667 0.220833 0.225 0.2375 0.241667 0.245833 0.25 0.266667 0.270833 0.275 0.279167 0.291667 0.295833 0.3 0.304167 0.316667 0.320833 0.325 0.333333 0.3375 0.341667 0.345833 0.3625 0.366667 0.370833 0.375 0.3875 0.391667 0.395833 0.4 0.4125 0.416667 0.420833 0.429167 0.433333 0.4375 0.441667 0.454167 0.458333 0.4625 0.470833 0.475 0.479167 0.4875 0.491667 0.495833 0.504167 0.508333 0.5125 0.520833 0.525 0.529167 0.5375 0.541667 0.545833 0.554167 0.558333 0.5625 0.570833 0.575 0.579167 0.5875 0.591667 0.595833 0.604167 0.608333 0.6125 0.620833 0.625 0.629167 0.6375 0.641667 0.645833 0.654167 0.658333 0.6625 0.670833 0.675 0.679167 0.6875 0.691667 0.695833 0.704167 0.708333 0.7125 0.720833 0.725 0.729167 0.7375 0.741667 0.745833 0.754167 0.758333 0.7625 0.770833 0.775 0.779167 0.795833 0.8 0.804167 0.808333 0.825 0.829167 0.833333 0.8375 0.845833 0.85 0.854167 0.8625 0.866667 0.870833 0.875 0.879167 0.883333 0.8875 0.891667 0.895833 0.9 0.904167 0.908333 0.9125 0.916667 0.920833 0.925 0.929167 0.933333 0.9375 0.941667 0.945833 0.95 0.954167 0.958333 0.9625 0.966667 0.970833 0.975 0.979167 0.983333 1 1 1 1 1 1
  line L10 (0.639, 6.5467) -> (0.5586, 5.7228)
  arc A5 (2.0935, 7.7212) -> (1.4639, 7.8649) centre (0, 0) ccw
  spline S5 degree 5 poles (1.4639, 7.8649) (1.4593, 7.8604) (1.4532, 7.8543) (1.4456, 7.8467) (1.4365, 7.8376) (1.426, 7.8269) (1.4186, 7.8193) (1.4111, 7.8117) (1.4038, 7.8041) (1.3964, 7.7965) (1.3891, 7.7889) (1.3818, 7.7813) (1.3746, 7.7738) (1.3674, 7.7662) (1.3602, 7.7586) (1.3531, 7.751) (1.346, 7.7434) (1.3389, 7.7359) (1.3319, 7.7283) (1.3249, 7.7207) (1.318, 7.7132) (1.311, 7.7056) (1.3042, 7.698) (1.2973, 7.6905) (1.2905, 7.6829) (1.2838, 7.6754) (1.2771, 7.6678) (1.2704, 7.6603) (1.2637, 7.6528) (1.2571, 7.6452) (1.2492, 7.6362) (1.2414, 7.6272) (1.2336, 7.6182) (1.2259, 7.6092) (1.2156, 7.5972) (1.2068, 7.5867) (1.198, 7.5763) (1.1893, 7.5658) (1.1782, 7.5524) (1.1696, 7.542) (1.1611, 7.5316) (1.1527, 7.5212) (1.142, 7.5079) (1.1338, 7.4975) (1.1256, 7.4872) (1.1163, 7.4754) (1.1072, 7.4636) (1.1004, 7.4548) (1.0925, 7.4446) (1.0847, 7.4343) (1.0781, 7.4256) (1.0705, 7.4154) (1.0629, 7.4052) (1.0564, 7.3965) (1.049, 7.3864) (1.0416, 7.3763) (1.0353, 7.3676) (1.0281, 7.3576) (1.0209, 7.3475) (1.0148, 7.339) (1.0078, 7.329) (1.0008, 7.319) (0.9949, 7.3105) (0.9881, 7.3006) (0.9813, 7.2907) (0.9756, 7.2823) (0.969, 7.2724) (0.9624, 7.2626) (0.9569, 7.2543) (0.9504, 7.2445) (0.9441, 7.2348) (0.9387, 7.2265) (0.9325, 7.2169) (0.9263, 7.2073) (0.9211, 7.199) (0.9151, 7.1895) (0.9092, 7.18) (0.9042, 7.1719) (0.8984, 7.1624) (0.8926, 7.153) (0.8878, 7.145) (0.8822, 7.1356) (0.8766, 7.1263) (0.8719, 7.1184) (0.8665, 7.1092) (0.8612, 7.1) (0.8567, 7.0922) (0.8515, 7.0831) (0.8464, 7.074) (0.842, 7.0663) (0.837, 7.0573) (0.8321, 7.0484) (0.8279, 7.0408) (0.8231, 7.0319) (0.8184, 7.0231) (0.8144, 7.0156) (0.8098, 7.0069) (0.8053, 6.9983) (0.8014, 6.9909) (0.797, 6.9823) (0.7927, 6.9738) (0.789, 6.9666) (0.7848, 6.9582) (0.7807, 6.9498) (0.7772, 6.9427) (0.7732, 6.9344) (0.7692, 6.9262) (0.7659, 6.9193) (0.7615, 6.91) (0.7572, 6.9008) (0.7536, 6.8929) (0.7499, 6.885) (0.7454, 6.8749) (0.7419, 6.8672) (0.7386, 6.8595) (0.7352, 6.8519) (0.7306, 6.8411) (0.727, 6.8326) (0.7234, 6.8242) (0.72, 6.8158) (0.7158, 6.8055) (0.7129, 6.7984) (0.7101, 6.7914) (0.7074, 6.7844) (0.704, 6.7755) (0.7014, 6.7687) (0.6988, 6.762) (0.696, 6.7544) (0.6933, 6.7469) (0.6913, 6.7414) (0.689, 6.735) (0.6868, 6.7286) (0.6849, 6.7233) (0.6828, 6.7171) (0.6807, 6.7111) (0.679, 6.7059) (0.6771, 6.7) (0.6752, 6.6942) (0.6736, 6.6893) (0.6718, 6.6836) (0.6701, 6.678) (0.6686, 6.6734) (0.667, 6.668) (0.6654, 6.6627) (0.6641, 6.6582) (0.6626, 6.6531) (0.6612, 6.6481) (0.66, 6.6439) (0.6587, 6.639) (0.6574, 6.6343) (0.6563, 6.6303) (0.6553, 6.6265) (0.654, 6.6214) (0.6529, 6.6171) (0.6519, 6.6129) (0.6509, 6.6088) (0.65, 6.6048) (0.6493, 6.6021) (0.6487, 6.5994) (0.6481, 6.5967) (0.6475, 6.5941) (0.6469, 6.5916) (0.6464, 6.5891) (0.6459, 6.5867) (0.6454, 6.5844) (0.6449, 6.5821) (0.6445, 6.5799) (0.6441, 6.5777) (0.6437, 6.5756) (0.6433, 6.5736) (0.6429, 6.5717) (0.6425, 6.5698) (0.6422, 6.568) (0.6419, 6.5662) (0.6416, 6.5645) (0.6413, 6.5629) (0.6411, 6.5614) (0.6408, 6.5599) (0.6406, 6.5585) (0.6404, 6.5572) (0.6402, 6.556) (0.64, 6.5548) (0.6399, 6.5537) (0.6397, 6.5527) (0.6396, 6.5517) (0.6395, 6.5509) (0.6394, 6.5501) (0.6393, 6.5494) (0.6392, 6.5486) (0.6391, 6.5481) (0.6391, 6.5478) (0.6391, 6.5475) (0.6391, 6.5474) knots -1 -1 -1 -1 -1 -1 -0.9875 -0.983333 -0.979167 -0.975 -0.970833 -0.966667 -0.9625 -0.958333 -0.954167 -0.95 -0.945833 -0.941667 -0.9375 -0.933333 -0.929167 -0.925 -0.920833 -0.916667 -0.9125 -0.908333 -0.904167 -0.9 -0.895833 -0.891667 -0.8875 -0.883333 -0.879167 -0.875 -0.870833 -0.8625 -0.858333 -0.854167 -0.85 -0.8375 -0.833333 -0.829167 -0.825 -0.8125 -0.808333 -0.804167 -0.8 -0.7875 -0.783333 -0.779167 -0.770833 -0.766667 -0.7625 -0.754167 -0.75 -0.745833 -0.7375 -0.733333 -0.729167 -0.720833 -0.716667 -0.7125 -0.704167 -0.7 -0.695833 -0.6875 -0.683333 -0.679167 -0.670833 -0.666667 -0.6625 -0.654167 -0.65 -0.645833 -0.6375 -0.633333 -0.629167 -0.620833 -0.616667 -0.6125 -0.604167 -0.6 -0.595833 -0.5875 -0.583333 -0.579167 -0.570833 -0.566667 -0.5625 -0.554167 -0.55 -0.545833 -0.5375 -0.533333 -0.529167 -0.520833 -0.516667 -0.5125 -0.504167 -0.5 -0.495833 -0.4875 -0.483333 -0.479167 -0.470833 -0.466667 -0.4625 -0.454167 -0.45 -0.445833 -0.4375 -0.433333 -0.429167 -0.416667 -0.4125 -0.408333 -0.404167 -0.391667 -0.3875 -0.383333 -0.379167 -0.3625 -0.358333 -0.354167 -0.35 -0.3375 -0.333333 -0.329167 -0.325 -0.3125 -0.308333 -0.304167 -0.295833 -0.291667 -0.2875 -0.279167 -0.275 -0.270833 -0.2625 -0.258333 -0.254167 -0.245833 -0.241667 -0.2375 -0.229167 -0.225 -0.220833 -0.2125 -0.208333 -0.204167 -0.195833 -0.191667 -0.1875 -0.179167 -0.175 -0.170833 -0.166667 -0.154167 -0.15 -0.145833 -0.141667 -0.1375 -0.133333 -0.129167 -0.125 -0.120833 -0.116667 -0.1125 -0.108333 -0.104167 -0.1 -0.095833 -0.091667 -0.0875 -0.083333 -0.079167 -0.075 -0.070833 -0.066667 -0.0625 -0.058333 -0.054167 -0.05 -0.045833 -0.041667 -0.0375 -0.033333 -0.029167 -0.025 -0.020833 -0.016667 -0.0125 -0.008333 0 0 0 0 0 0
  line L11 (3.4162, 5.6212) -> (2.9863, 4.9137)
  line L12 (-2.265, 6.1763) -> (-2.2648, 6.1757)
  spline S6 degree 5 poles (-2.0935, 7.7212) (-2.0957, 7.7151) (-2.0986, 7.707) (-2.1021, 7.6968) (-2.1063, 7.6847) (-2.1112, 7.6705) (-2.1146, 7.6605) (-2.118, 7.6504) (-2.1213, 7.6403) (-2.1247, 7.6303) (-2.128, 7.6203) (-2.1312, 7.6103) (-2.1345, 7.6003) (-2.1377, 7.5904) (-2.1408, 7.5804) (-2.144, 7.5705) (-2.1471, 7.5606) (-2.1501, 7.5507) (-2.1532, 7.5408) (-2.1562, 7.531) (-2.1592, 7.5211) (-2.1621, 7.5113) (-2.165, 7.5015) (-2.1679, 7.4918) (-2.1708, 7.482) (-2.1736, 7.4723) (-2.1764, 7.4626) (-2.1791, 7.4529) (-2.1818, 7.4432) (-2.1845, 7.4336) (-2.1877, 7.422) (-2.1909, 7.4105) (-2.194, 7.399) (-2.197, 7.3875) (-2.2011, 7.3723) (-2.2045, 7.359) (-2.2079, 7.3458) (-2.2112, 7.3326) (-2.2154, 7.3157) (-2.2186, 7.3026) (-2.2217, 7.2895) (-2.2248, 7.2765) (-2.2291, 7.258) (-2.2324, 7.2433) (-2.2357, 7.2286) (-2.2388, 7.214) (-2.2427, 7.1958) (-2.2454, 7.1832) (-2.248, 7.1706) (-2.2505, 7.158) (-2.2537, 7.1419) (-2.2561, 7.1295) (-2.2584, 7.1171) (-2.2607, 7.1048) (-2.2639, 7.0872) (-2.2664, 7.0733) (-2.2688, 7.0594) (-2.2711, 7.0456) (-2.2739, 7.0284) (-2.2758, 7.0165) (-2.2776, 7.0046) (-2.2794, 6.9928) (-2.2817, 6.9777) (-2.2833, 6.966) (-2.285, 6.9543) (-2.2868, 6.9411) (-2.2885, 6.928) (-2.2897, 6.9182) (-2.2911, 6.9068) (-2.2925, 6.8954) (-2.2936, 6.8858) (-2.2949, 6.8746) (-2.2961, 6.8634) (-2.2971, 6.8539) (-2.2983, 6.8429) (-2.2993, 6.8319) (-2.3002, 6.8226) (-2.3012, 6.8117) (-2.3022, 6.801) (-2.303, 6.7918) (-2.3038, 6.7811) (-2.3046, 6.7706) (-2.3053, 6.7615) (-2.3061, 6.7511) (-2.3067, 6.7407) (-2.3073, 6.7318) (-2.3079, 6.7216) (-2.3085, 6.7114) (-2.3089, 6.7027) (-2.3094, 6.6927) (-2.3099, 6.6827) (-2.3102, 6.6742) (-2.3106, 6.6644) (-2.3109, 6.6546) (-2.3112, 6.6463) (-2.3114, 6.6367) (-2.3116, 6.6271) (-2.3118, 6.619) (-2.3119, 6.6096) (-2.312, 6.6003) (-2.3121, 6.5923) (-2.3121, 6.5832) (-2.3121, 6.5741) (-2.3121, 6.5663) (-2.3121, 6.5574) (-2.312, 6.5485) (-2.3118, 6.541) (-2.3117, 6.5323) (-2.3115, 6.5237) (-2.3113, 6.5163) (-2.3111, 6.5078) (-2.3108, 6.4995) (-2.3105, 6.4924) (-2.3102, 6.4841) (-2.3098, 6.476) (-2.3095, 6.4691) (-2.309, 6.4611) (-2.3086, 6.4532) (-2.3082, 6.4466) (-2.3077, 6.4388) (-2.3072, 6.4312) (-2.3067, 6.4248) (-2.3061, 6.4173) (-2.3055, 6.41) (-2.305, 6.4038) (-2.3044, 6.3966) (-2.3037, 6.3895) (-2.3031, 6.3835) (-2.3025, 6.3766) (-2.3017, 6.3698) (-2.3011, 6.3641) (-2.3004, 6.3575) (-2.2996, 6.3509) (-2.299, 6.3454) (-2.2982, 6.3391) (-2.2974, 6.3329) (-2.2967, 6.3277) (-2.2958, 6.3216) (-2.295, 6.3157) (-2.2943, 6.3107) (-2.2934, 6.305) (-2.2926, 6.2994) (-2.2918, 6.2947) (-2.2909, 6.2893) (-2.2901, 6.284) (-2.2893, 6.2795) (-2.2884, 6.2744) (-2.2875, 6.2695) (-2.2867, 6.2653) (-2.286, 6.2612) (-2.2852, 6.2572) (-2.2843, 6.2526) (-2.2834, 6.2482) (-2.2825, 6.2439) (-2.2816, 6.2397) (-2.2808, 6.2356) (-2.2801, 6.2328) (-2.2795, 6.23) (-2.2789, 6.2273) (-2.2783, 6.2246) (-2.2777, 6.222) (-2.2771, 6.2195) (-2.2765, 6.2171) (-2.2759, 6.2147) (-2.2754, 6.2123) (-2.2748, 6.2101) (-2.2742, 6.2079) (-2.2737, 6.2058) (-2.2732, 6.2037) (-2.2726, 6.2017) (-2.2721, 6.1998) (-2.2716, 6.198) (-2.2711, 6.1962) (-2.2706, 6.1945) (-2.2702, 6.1928) (-2.2697, 6.1913) (-2.2693, 6.1898) (-2.2689, 6.1883) (-2.2685, 6.187) (-2.2681, 6.1857) (-2.2677, 6.1845) (-2.2674, 6.1834) (-2.267, 6.1823) (-2.2667, 6.1813) (-2.2664, 6.1804) (-2.2662, 6.1796) (-2.2659, 6.1788) (-2.2657, 6.1782) (-2.2654, 6.1774) (-2.2653, 6.1769) (-2.2652, 6.1766) (-2.2651, 6.1764) (-2.265, 6.1763) knots -1 -1 -1 -1 -1 -1 -0.9875 -0.983333 -0.979167 -0.975 -0.970833 -0.966667 -0.9625 -0.958333 -0.954167 -0.95 -0.945833 -0.941667 -0.9375 -0.933333 -0.929167 -0.925 -0.920833 -0.916667 -0.9125 -0.908333 -0.904167 -0.9 -0.895833 -0.891667 -0.8875 -0.883333 -0.879167 -0.875 -0.870833 -0.8625 -0.858333 -0.854167 -0.85 -0.8375 -0.833333 -0.829167 -0.825 -0.8125 -0.808333 -0.804167 -0.8 -0.783333 -0.779167 -0.775 -0.770833 -0.758333 -0.754167 -0.75 -0.745833 -0.733333 -0.729167 -0.725 -0.720833 -0.704167 -0.7 -0.695833 -0.691667 -0.679167 -0.675 -0.670833 -0.666667 -0.654167 -0.65 -0.645833 -0.6375 -0.633333 -0.629167 -0.620833 -0.616667 -0.6125 -0.604167 -0.6 -0.595833 -0.5875 -0.583333 -0.579167 -0.570833 -0.566667 -0.5625 -0.554167 -0.55 -0.545833 -0.5375 -0.533333 -0.529167 -0.520833 -0.516667 -0.5125 -0.504167 -0.5 -0.495833 -0.4875 -0.483333 -0.479167 -0.470833 -0.466667 -0.4625 -0.454167 -0.45 -0.445833 -0.4375 -0.433333 -0.429167 -0.420833 -0.416667 -0.4125 -0.404167 -0.4 -0.395833 -0.3875 -0.383333 -0.379167 -0.370833 -0.366667 -0.3625 -0.354167 -0.35 -0.345833 -0.3375 -0.333333 -0.329167 -0.320833 -0.316667 -0.3125 -0.304167 -0.3 -0.295833 -0.2875 -0.283333 -0.279167 -0.270833 -0.266667 -0.2625 -0.254167 -0.25 -0.245833 -0.2375 -0.233333 -0.229167 -0.220833 -0.216667 -0.2125 -0.204167 -0.2 -0.195833 -0.1875 -0.183333 -0.179167 -0.175 -0.170833 -0.158333 -0.154167 -0.15 -0.145833 -0.141667 -0.1375 -0.133333 -0.129167 -0.125 -0.120833 -0.116667 -0.1125 -0.108333 -0.104167 -0.1 -0.095833 -0.091667 -0.0875 -0.083333 -0.079167 -0.075 -0.070833 -0.066667 -0.0625 -0.058333 -0.054167 -0.05 -0.045833 -0.041667 -0.0375 -0.033333 -0.029167 -0.025 -0.020833 -0.016667 -0.0125 -0.008333 0 0 0 0 0 0
  line L13 (-0.639, 6.5467) -> (-0.6391, 6.5474)
  line L14 (-0.5586, 5.7228) -> (-0.639, 6.5467)
  arc A6 (0.5586, 5.7228) -> (-0.5586, 5.7228) centre (0, 0) ccw
  spline S7 degree 5 poles (-0.6391, 6.5474) (-0.6391, 6.5475) (-0.6391, 6.5476) (-0.6391, 6.5478) (-0.6391, 6.5482) (-0.6392, 6.5488) (-0.6393, 6.5494) (-0.6394, 6.5501) (-0.6395, 6.5509) (-0.6396, 6.5517) (-0.6397, 6.5527) (-0.6399, 6.5537) (-0.64, 6.5548) (-0.6402, 6.556) (-0.6404, 6.5572) (-0.6406, 6.5585) (-0.6408, 6.5599) (-0.6411, 6.5614) (-0.6413, 6.5629) (-0.6416, 6.5645) (-0.6419, 6.5662) (-0.6422, 6.568) (-0.6425, 6.5698) (-0.6429, 6.5717) (-0.6433, 6.5736) (-0.6437, 6.5756) (-0.6441, 6.5777) (-0.6445, 6.5799) (-0.6449, 6.5821) (-0.6454, 6.5844) (-0.6459, 6.5867) (-0.6464, 6.5891) (-0.6469, 6.5916) (-0.6475, 6.5941) (-0.6481, 6.5967) (-0.6488, 6.5999) (-0.6496, 6.6032) (-0.6504, 6.6065) (-0.6515, 6.6111) (-0.6529, 6.6171) (-0.6543, 6.6226) (-0.6558, 6.6284) (-0.6574, 6.6343) (-0.6592, 6.6411) (-0.6608, 6.6466) (-0.6624, 6.6523) (-0.6641, 6.6582) (-0.6663, 6.6657) (-0.6679, 6.671) (-0.6696, 6.6765) (-0.6713, 6.682) (-0.6738, 6.6901) (-0.676, 6.6966) (-0.6781, 6.7034) (-0.6804, 6.7102) (-0.6834, 6.7189) (-0.6855, 6.7251) (-0.6877, 6.7313) (-0.69, 6.7377) (-0.6929, 6.746) (-0.6953, 6.7525) (-0.6978, 6.7591) (-0.7003, 6.7658) (-0.704, 6.7755) (-0.707, 6.7834) (-0.7101, 6.7913) (-0.7133, 6.7994) (-0.7175, 6.8096) (-0.7204, 6.8169) (-0.7234, 6.8242) (-0.7265, 6.8315) (-0.7306, 6.8411) (-0.7338, 6.8486) (-0.7371, 6.8562) (-0.7405, 6.8639) (-0.7454, 6.8749) (-0.7494, 6.8839) (-0.7535, 6.8929) (-0.7578, 6.902) (-0.7631, 6.9135) (-0.767, 6.9216) (-0.7709, 6.9297) (-0.7749, 6.938) (-0.7801, 6.9486) (-0.7842, 6.957) (-0.7884, 6.9654) (-0.7927, 6.9738) (-0.7983, 6.9848) (-0.8027, 6.9933) (-0.8072, 7.002) (-0.8118, 7.0106) (-0.8184, 7.0231) (-0.8238, 7.0332) (-0.8293, 7.0433) (-0.8349, 7.0535) (-0.842, 7.0663) (-0.8471, 7.0753) (-0.8522, 7.0844) (-0.8574, 7.0935) (-0.865, 7.1066) (-0.8712, 7.1171) (-0.8774, 7.1277) (-0.8837, 7.1383) (-0.891, 7.1503) (-0.8959, 7.1584) (-0.9008, 7.1665) (-0.9067, 7.1759) (-0.9126, 7.1854) (-0.9177, 7.1936) (-0.9237, 7.2031) (-0.9298, 7.2127) (-0.9351, 7.221) (-0.9414, 7.2307) (-0.9477, 7.2404) (-0.9532, 7.2487) (-0.9596, 7.2584) (-0.9661, 7.2682) (-0.9718, 7.2766) (-0.9784, 7.2865) (-0.9852, 7.2963) (-0.991, 7.3048) (-0.9979, 7.3147) (-1.0048, 7.3247) (-1.0108, 7.3333) (-1.0179, 7.3432) (-1.025, 7.3533) (-1.0312, 7.3619) (-1.0385, 7.372) (-1.0458, 7.3821) (-1.0522, 7.3907) (-1.0596, 7.4009) (-1.0672, 7.411) (-1.0737, 7.4198) (-1.0814, 7.43) (-1.0892, 7.4402) (-1.0959, 7.449) (-1.1038, 7.4592) (-1.1118, 7.4695) (-1.1187, 7.4783) (-1.1268, 7.4887) (-1.1349, 7.499) (-1.142, 7.5079) (-1.1503, 7.5182) (-1.1587, 7.5286) (-1.166, 7.5375) (-1.1769, 7.5509) (-1.188, 7.5643) (-1.198, 7.5763) (-1.208, 7.5882) (-1.2195, 7.6017) (-1.2284, 7.6122) (-1.2375, 7.6227) (-1.2466, 7.6332) (-1.2558, 7.6437) (-1.2637, 7.6528) (-1.2704, 7.6603) (-1.2771, 7.6678) (-1.2838, 7.6754) (-1.2905, 7.6829) (-1.2973, 7.6905) (-1.3042, 7.698) (-1.311, 7.7056) (-1.318, 7.7132) (-1.3249, 7.7207) (-1.3319, 7.7283) (-1.3389, 7.7359) (-1.346, 7.7434) (-1.3531, 7.751) (-1.3602, 7.7586) (-1.3674, 7.7662) (-1.3746, 7.7738) (-1.3818, 7.7813) (-1.3891, 7.7889) (-1.3964, 7.7965) (-1.4038, 7.8041) (-1.4111, 7.8117) (-1.4186, 7.8193) (-1.4305, 7.8315) (-1.4411, 7.8421) (-1.4502, 7.8512) (-1.4578, 7.8588) (-1.4639, 7.8649) knots 0 0 0 0 0 0 0.004167 0.008333 0.0125 0.016667 0.020833 0.025 0.029167 0.033333 0.0375 0.041667 0.045833 0.05 0.054167 0.058333 0.0625 0.066667 0.070833 0.075 0.079167 0.083333 0.0875 0.091667 0.095833 0.1 0.104167 0.108333 0.1125 0.116667 0.120833 0.125 0.129167 0.133333 0.1375 0.141667 0.15 0.154167 0.158333 0.170833 0.183333 0.1875 0.191667 0.195833 0.2125 0.216667 0.220833 0.225 0.2375 0.241667 0.245833 0.25 0.266667 0.270833 0.275 0.279167 0.291667 0.295833 0.3 0.304167 0.316667 0.320833 0.325 0.329167 0.345833 0.35 0.354167 0.358333 0.370833 0.375 0.379167 0.383333 0.395833 0.4 0.404167 0.408333 0.425 0.429167 0.433333 0.4375 0.45 0.454167 0.458333 0.4625 0.475 0.479167 0.483333 0.4875 0.5 0.504167 0.508333 0.5125 0.529167 0.533333 0.5375 0.541667 0.554167 0.558333 0.5625 0.566667 0.583333 0.5875 0.591667 0.595833 0.604167 0.608333 0.6125 0.620833 0.625 0.629167 0.6375 0.641667 0.645833 0.654167 0.658333 0.6625 0.670833 0.675 0.679167 0.6875 0.691667 0.695833 0.704167 0.708333 0.7125 0.720833 0.725 0.729167 0.7375 0.741667 0.745833 0.754167 0.758333 0.7625 0.770833 0.775 0.779167 0.7875 0.791667 0.795833 0.804167 0.808333 0.8125 0.820833 0.825 0.829167 0.845833 0.85 0.854167 0.858333 0.866667 0.875 0.879167 0.883333 0.8875 0.891667 0.895833 0.9 0.904167 0.908333 0.9125 0.916667 0.920833 0.925 0.929167 0.933333 0.9375 0.941667 0.945833 0.95 0.954167 0.958333 0.9625 0.966667 0.970833 0.975 0.979167 0.983333 1 1 1 1 1 1
  arc A7 (-1.4639, 7.8649) -> (-2.0935, 7.7212) centre (0, 0) ccw
  line L15 (-6.5248, 0.8338) -> (-6.5254, 0.8339)
  line L16 (-5.7036, 0.7289) -> (-6.5248, 0.8338)
  arc A8 (-5.455, 1.818) -> (-5.7036, 0.7289) centre (0, 0) ccw
  spline S8 degree 5 poles (-6.5254, 0.8339) (-6.5255, 0.8339) (-6.5256, 0.8339) (-6.5259, 0.834) (-6.5263, 0.834) (-6.5268, 0.834) (-6.5274, 0.8341) (-6.5281, 0.8342) (-6.5289, 0.8343) (-6.5298, 0.8343) (-6.5307, 0.8344) (-6.5318, 0.8345) (-6.5329, 0.8346) (-6.5341, 0.8347) (-6.5353, 0.8348) (-6.5366, 0.8349) (-6.5381, 0.8349) (-6.5395, 0.835) (-6.5411, 0.8351) (-6.5427, 0.8352) (-6.5444, 0.8353) (-6.5462, 0.8354) (-6.548, 0.8355) (-6.55, 0.8356) (-6.5519, 0.8356) (-6.554, 0.8357) (-6.5561, 0.8358) (-6.5583, 0.8358) (-6.5606, 0.8359) (-6.5629, 0.8359) (-6.5653, 0.836) (-6.5678, 0.836) (-6.5703, 0.836) (-6.5729, 0.8361) (-6.5755, 0.8361) (-6.5788, 0.8361) (-6.5821, 0.8361) (-6.5856, 0.836) (-6.5903, 0.836) (-6.5964, 0.8359) (-6.6022, 0.8358) (-6.6081, 0.8356) (-6.6149, 0.8353) (-6.6206, 0.8351) (-6.6249, 0.8349) (-6.6293, 0.8347) (-6.6352, 0.8344) (-6.6406, 0.8341) (-6.646, 0.8337) (-6.6524, 0.8333) (-6.6589, 0.8328) (-6.6639, 0.8324) (-6.6697, 0.832) (-6.6757, 0.8314) (-6.6809, 0.831) (-6.6871, 0.8304) (-6.6934, 0.8298) (-6.6988, 0.8292) (-6.7053, 0.8286) (-6.7118, 0.8278) (-6.7175, 0.8272) (-6.7242, 0.8264) (-6.731, 0.8256) (-6.737, 0.8248) (-6.7439, 0.8239) (-6.751, 0.823) (-6.7571, 0.8221) (-6.7644, 0.8211) (-6.7717, 0.82) (-6.778, 0.8191) (-6.7855, 0.8179) (-6.7931, 0.8167) (-6.7996, 0.8156) (-6.8074, 0.8144) (-6.8152, 0.813) (-6.8219, 0.8118) (-6.8299, 0.8104) (-6.8379, 0.809) (-6.8449, 0.8077) (-6.8531, 0.8061) (-6.8613, 0.8045) (-6.8685, 0.8031) (-6.8769, 0.8014) (-6.8853, 0.7997) (-6.8927, 0.7981) (-6.9013, 0.7963) (-6.91, 0.7944) (-6.9175, 0.7927) (-6.9263, 0.7907) (-6.9352, 0.7887) (-6.9428, 0.7869) (-6.9519, 0.7848) (-6.9609, 0.7826) (-6.9688, 0.7806) (-6.978, 0.7783) (-6.9873, 0.776) (-6.9953, 0.7739) (-7.0047, 0.7715) (-7.0142, 0.769) (-7.0223, 0.7668) (-7.0319, 0.7642) (-7.0415, 0.7615) (-7.0499, 0.7591) (-7.0596, 0.7564) (-7.0694, 0.7535) (-7.0779, 0.7511) (-7.0878, 0.7481) (-7.0978, 0.7451) (-7.1064, 0.7425) (-7.1165, 0.7394) (-7.1267, 0.7362) (-7.1354, 0.7334) (-7.1457, 0.7302) (-7.156, 0.7268) (-7.1649, 0.7239) (-7.1753, 0.7205) (-7.1857, 0.7169) (-7.1947, 0.7139) (-7.2053, 0.7103) (-7.2159, 0.7066) (-7.225, 0.7034) (-7.2357, 0.6996) (-7.2465, 0.6957) (-7.2558, 0.6923) (-7.2666, 0.6883) (-7.2775, 0.6843) (-7.2869, 0.6808) (-7.2978, 0.6766) (-7.3089, 0.6724) (-7.3183, 0.6687) (-7.3295, 0.6644) (-7.3406, 0.66) (-7.3502, 0.6561) (-7.3614, 0.6516) (-7.3727, 0.647) (-7.3824, 0.643) (-7.3937, 0.6383) (-7.4051, 0.6335) (-7.4149, 0.6294) (-7.4264, 0.6245) (-7.4379, 0.6195) (-7.4478, 0.6152) (-7.4594, 0.6101) (-7.471, 0.605) (-7.481, 0.6005) (-7.4927, 0.5952) (-7.5044, 0.5899) (-7.5145, 0.5853) (-7.5263, 0.5798) (-7.5381, 0.5743) (-7.5482, 0.5695) (-7.5584, 0.5646) (-7.5703, 0.5589) (-7.5806, 0.554) (-7.5908, 0.549) (-7.6028, 0.5431) (-7.6149, 0.5371) (-7.6252, 0.5319) (-7.6373, 0.5259) (-7.6494, 0.5197) (-7.6598, 0.5144) (-7.6703, 0.509) (-7.6842, 0.5017) (-7.6964, 0.4953) (-7.7087, 0.4888) (-7.721, 0.4823) (-7.7333, 0.4756) (-7.7421, 0.4709) (-7.7509, 0.4661) (-7.7598, 0.4612) (-7.7686, 0.4563) (-7.7775, 0.4514) (-7.7863, 0.4465) (-7.7952, 0.4415) (-7.8041, 0.4365) (-7.813, 0.4314) (-7.822, 0.4263) (-7.8309, 0.4212) (-7.8398, 0.4161) (-7.8488, 0.4109) (-7.8578, 0.4056) (-7.8667, 0.4004) (-7.8757, 0.3951) (-7.8847, 0.3897) (-7.8937, 0.3843) (-7.9028, 0.3789) (-7.9118, 0.3735) (-7.9208, 0.368) (-7.9299, 0.3625) (-7.9389, 0.357) (-7.9534, 0.348) (-7.9662, 0.3401) (-7.9771, 0.3333) (-7.9862, 0.3275) (-7.9935, 0.3229) knots 0 0 0 0 0 0 0.004167 0.008333 0.0125 0.016667 0.020833 0.025 0.029167 0.033333 0.0375 0.041667 0.045833 0.05 0.054167 0.058333 0.0625 0.066667 0.070833 0.075 0.079167 0.083333 0.0875 0.091667 0.095833 0.1 0.104167 0.108333 0.1125 0.116667 0.120833 0.125 0.129167 0.133333 0.1375 0.141667 0.15 0.154167 0.158333 0.170833 0.183333 0.1875 0.191667 0.2 0.204167 0.208333 0.2125 0.225 0.229167 0.233333 0.241667 0.245833 0.25 0.258333 0.2625 0.266667 0.275 0.279167 0.283333 0.291667 0.295833 0.3 0.308333 0.3125 0.316667 0.325 0.329167 0.333333 0.341667 0.345833 0.35 0.358333 0.3625 0.366667 0.375 0.379167 0.383333 0.391667 0.395833 0.4 0.408333 0.4125 0.416667 0.425 0.429167 0.433333 0.441667 0.445833 0.45 0.458333 0.4625 0.466667 0.475 0.479167 0.483333 0.491667 0.495833 0.5 0.508333 0.5125 0.516667 0.525 0.529167 0.533333 0.541667 0.545833 0.55 0.558333 0.5625 0.566667 0.575 0.579167 0.583333 0.591667 0.595833 0.6 0.608333 0.6125 0.616667 0.625 0.629167 0.633333 0.641667 0.645833 0.65 0.658333 0.6625 0.666667 0.675 0.679167 0.683333 0.691667 0.695833 0.7 0.708333 0.7125 0.716667 0.725 0.729167 0.733333 0.741667 0.745833 0.75 0.758333 0.7625 0.766667 0.775 0.779167 0.783333 0.791667 0.795833 0.8 0.804167 0.8125 0.816667 0.820833 0.829167 0.833333 0.8375 0.845833 0.85 0.854167 0.858333 0.870833 0.875 0.879167 0.883333 0.8875 0.891667 0.895833 0.9 0.904167 0.908333 0.9125 0.916667 0.920833 0.925 0.929167 0.933333 0.9375 0.941667 0.945833 0.95 0.954167 0.958333 0.9625 0.966667 0.970833 0.975 0.979167 0.983333 1 1 1 1 1 1
  line L17 (-6.5248, -0.8338) -> (-5.7036, -0.7289)
  line L18 (-6.5254, -0.8339) -> (-6.5248, -0.8338)
  arc A9 (-5.7036, -0.7289) -> (-5.455, -1.818) centre (0, 0) ccw
  arc A10 (-7.9935, 0.3229) -> (-7.9935, -0.3229) centre (0, 0) ccw